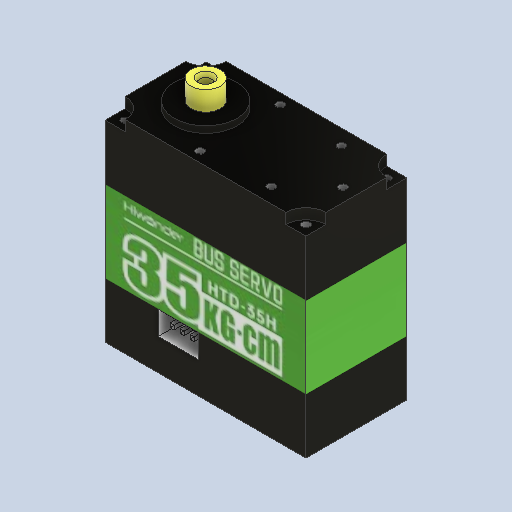
# Autodesk Inventor part: HTD-35H Servo
Saved by Autodesk Inventor 2023 (Build 270158000, 158)
## iProperties
Created: 2022-09-17
Part Number: HTD-35H Servo
Material: 일반
Document SubType Name: Modeling
Designer: 박동준
Density: 1 g/cm^3
Appearance: 기본값
Sheet Metal Rule: Default
품번: 6
Author: 박동준
Autodesk Inventor part; units mm, degrees
sketch "스케치1" plane through (0, 0, 0) normal (0, 0, 1) x (1, 0, 0)
  line L0 (-20.05, 20.25) -> (20.05, 20.25)
  line L1 (20.05, 20.25) -> (20.05, -20.25)
  line L2 (20.05, -20.25) -> (-20.05, -20.25)
  line L3 (-20.05, -20.25) -> (-20.05, 20.25)
  point P0 (0, 0)
  point P1 (0, 20.25)
  point P2 (-20.05, 0)
  dimension "d0" = 40.5
  dimension "d1" = 40.1
  constraints: 8 end point, 2 midpoint, 2 parallel, 1 horizontal, 1 horizontal alignment, 1 perpendicular, 1 vertical alignment
  measures "d0" distance of L2.end L0.start
  measures "d1" distance of L0.start L0.end
extrude "돌출1" add sketch "스케치1" along normal mid plane 20.14
sketch "스케치2" plane through (-20.05, 20.25, 10.07) normal (0, 1, 0) x (1, 0, 0)
  line L0 (16.9, 18.07) -> (16.9, 2.07) construction
  line L1 (0, 0) -> (40.1, 0) projected
  circle A0 centre (10, 10.07) radius 6.25
  line L2 (0, 20.14) -> (0, 0) projected
  point P0 (20.05, 10.07)
  point P1 (30.0912, 5.5667)
  point P2 (30.1, 12.7989)
  point P3 (37.0706, 12.5174)
  point P4 (16.9, 10.07)
  dimension "d4" = 16
  dimension "d6" = 13.2
  dimension "d7" = 12.5
  dimension "d8" = 6.9
  dimension "d9" = 10
  constraints: 2 end point, 2 horizontal alignment, 1 centre point, 1 midpoint, 1 perpendicular, 1 vertical alignment
  measures "d4" distance of L0.end L0.start
  measures "d6" horizontal distance of point (30.1, 12.799) L0.start
  measures "d7" diameter of A0
  measures "d8" horizontal distance of L0.start A0.centre
  measures "d9" distance from line of A0.centre L2
extrude "돌출2" add sketch "스케치2" along normal blind 1.3
sketch "스케치3" plane through (-20.05, -20.25, 10.07) normal (0, -1, 0) x (1, 0, 0)
  circle A0 centre (10, -10.07) radius 6.35
  line L0 (0, 0) -> (0, -20.14) projected
  point P0 (20.05, -10.07)
  dimension "d12" = 12.7
  dimension "d13" = 10
  constraints: 1 centre point, 1 horizontal alignment
  measures "d12" diameter of A0
  measures "d13" distance from line of A0.centre L0
extrude "돌출3" add sketch "스케치3" along normal blind 1.6
sketch "스케치4" plane through (-20.05, -20.25, 10.07) normal (0, -1, 0) x (1, 0, 0)
  circle A0 centre (10, -10.07) radius 6.35 construction
  line L0 (40.1, -20.14) -> (40.1, 0) construction
  line L1 (0, 0) -> (40.1, 0) construction
  line L2 (0, 0) -> (0, -20.14) construction
  line L3 (40.1, -20.14) -> (0, -20.14) construction
  line L4 (2.5, -2.545) -> (2.5, -17.595) construction
  line L5 (22.5, -2.545) -> (22.5, -17.595) construction
  line L6 (37.6, -2.545) -> (37.6, -17.595) construction
  point P0 (20.05, -10.07)
  point P1 (2.5, -10.07)
  point P2 (22.5, -10.07)
  point P3 (37.6, -10.07)
  dimension "d16" = 15.05
  dimension "d17" = 20
  dimension "d18" = 15.1
  dimension "d19" = 2.5
  constraints: 6 end point, 3 horizontal alignment, 3 midpoint, 2 vertical, 1 perpendicular
  measures "d16" distance of L4.end L4.start
  measures "d17" distance of L5.end L4.end
  measures "d18" distance of L6.end L5.end
  measures "d19" distance from line of L2 L4.end
hole "구멍1" at (-17.55, -20.25, 7.525) at (-17.55, -20.25, -7.525) at (2.45, -20.25, -7.525) at (2.45, -20.25, 7.525) at (17.55, -20.25, 7.525) at (17.55, -20.25, -7.525) direction (0, 1, 0) diameter 1.567 depth 10.6 thread size "M2x0.4" class "6H" standard "ISO Metric profile"
sketch "스케치5" plane through (0, 0, 10.07) normal (0, 0, 1) x (1, 0, 0)
  line L0 (-9.45, -9.25) -> (-1.45, -9.25)
  line L1 (-1.45, -9.25) -> (-1.45, -13.95)
  line L2 (-1.45, -13.95) -> (-9.45, -13.95)
  line L3 (-9.45, -13.95) -> (-9.45, -9.25)
  line L4 (-20.05, -20.25) -> (20.05, -20.25) projected
  line L5 (20.05, -20.25) -> (20.05, 20.25) projected
  point P0 (0, 0)
  dimension "d27" = 8
  dimension "d28" = 11
  dimension "d37" = 4.7
  dimension "d38" = 21.5
  constraints: 8 end point, 2 parallel, 1 horizontal, 1 perpendicular
  measures "d27" distance of L1.end L2.end
  measures "d28" distance between parallel lines of L0 L4
  measures "d37" distance of L0.end L1.end
  measures "d38" distance between parallel lines of L5 L1
extrude "돌출4" cut sketch "스케치5" against normal blind 5
sketch "스케치6" plane through (-10.05, -21.85, 0) normal (0, -1, 0) x (1, 0, 0)
  circle A0 centre (0, 0) radius 6.35 projected
  circle A1 centre (0, 0) radius 3
  point P0 (10.05, 0)
  dimension "d31" = 6
  constraints: 1 centre point, 1 coincident
  measures "d31" diameter of A1
extrude "돌출5" add sketch "스케치6" along normal blind 4.3 contours A1
sketch "스케치7" plane through (-10.05, -26.15, 0) normal (0, -1, 0) x (1, 0, 0)
  circle A0 centre (0, 0) radius 3 projected
  circle A1 centre (0, 0) radius 1.5
  point P0 (10.05, 0)
  dimension "d34" = 3
  constraints: 1 centre point, 1 coincident
  measures "d34" diameter of A1
extrude "돌출6" cut sketch "스케치7" against normal blind 8 contours A1
sketch "스케치8" plane through (-20.05, -20.25, 10.07) normal (-1, 0, 0) x (0, 0, 1)
  line L0 (0, 0) -> (-20.14, 0) construction
  line L1 (0, 40.5) -> (0, 0) construction
  line L2 (-20.14, 40.5) -> (0, 40.5) construction
  line L3 (-20.14, 0) -> (-20.14, 40.5) construction
  line L4 (-14.07, 11) -> (-6.07, 11)
  line L5 (-6.07, 11) -> (-6.07, 6.3)
  line L6 (-6.07, 6.3) -> (-14.07, 6.3)
  line L7 (-14.07, 6.3) -> (-14.07, 11)
  point P0 (-10.07, 20.25)
  point P1 (-10.07, 11)
  dimension "d39" = 8
  dimension "d40" = 4.7
  dimension "d41" = 11
  constraints: 8 end point, 2 parallel, 1 horizontal, 1 midpoint, 1 perpendicular, 1 vertical alignment
  measures "d39" distance of L5.end L6.end
  measures "d40" distance of L4.end L5.end
  measures "d41" distance between parallel lines of L0 L4
extrude "돌출7" cut sketch "스케치8" against normal blind 5
sketch "스케치9" plane through (0, 0, -10.07) normal (0, 0, -1) x (-1, 0, 0)
  line L0 (1.45, -9.25) -> (9.45, -9.25)
  line L1 (9.45, -9.25) -> (9.45, -13.95)
  line L2 (9.45, -13.95) -> (1.45, -13.95)
  line L3 (1.45, -13.95) -> (1.45, -9.25)
  line L4 (-20.05, -20.25) -> (20.05, -20.25) projected
  line L5 (-20.05, 20.25) -> (-20.05, -20.25) projected
  point P0 (0, 0)
  dimension "d44" = 8
  dimension "d45" = 4.7
  dimension "d46" = 11
  dimension "d47" = 21.5
  constraints: 8 end point, 2 parallel, 1 horizontal, 1 perpendicular
  measures "d44" distance of L1.end L2.end
  measures "d45" distance of L0.end L1.end
  measures "d46" distance between parallel lines of L4 L0
  measures "d47" distance between parallel lines of L5 L3
extrude "돌출8" cut sketch "스케치9" against normal blind 5
sketch "스케치10" plane through (-20.05, 20.25, 10.07) normal (0, 1, 0) x (1, 0, 0)
  circle A0 centre (10, 10.07) radius 6.25 projected
  line L0 (16.9, 18.07) -> (16.9, 2.07) construction
  line L1 (30.12, 17.07) -> (30.12, 3.07) construction
  point P0 (20.05, 10.07)
  point P1 (37.42, 10.07)
  point P2 (16.9, 10.07)
  point P3 (30.12, 10.07)
  dimension "d50" = 6.9
  dimension "d51" = 13.22
  dimension "d52" = 16
  dimension "d53" = 7.3
  dimension "d165" = 14
  constraints: 4 end point, 3 horizontal alignment, 2 midpoint, 2 vertical, 2 vertical alignment
  measures "d50" horizontal distance of L0.start A0.centre
  measures "d51" horizontal distance of L1.start L0.start
  measures "d52" distance of L0.end L0.start
  measures "d53" horizontal distance of L1.start point (37.42, 10.07)
  measures "d165" distance of L1.end L1.start
sketch "스케치11" plane through (0, 0, 0) normal (0, 0, 1) x (1, 0, 0)
  line L0 (-3.8, 21.55) -> (-16.3, 21.55) projected
  line L1 (-16.3, 20.25) -> (-3.8, 20.25) projected
  line L2 (-3.8, 21.55) -> (-16.3, 21.55) projected
  line L3 (-10.05, 21.55) -> (-10.05, 26.55)
  line L4 (-8.85, 24.65) -> (-8.425, 25.45)
  line L5 (-8.425, 25.45) -> (-7.125, 25.45)
  line L6 (-7.125, 25.45) -> (-7.125, 21.55)
  line L7 (-8.85, 24.65) -> (-8.85, 21.55)
  line L8 (-8.85, 21.55) -> (-7.125, 21.55)
  point P0 (0, 0)
  dimension "d54" = 5
  dimension "d55" = 5.85
  dimension "d56" = 2.4
  dimension "d57" = 1.3
  dimension "d58" = 0.8
  dimension "d59" = 3.9
  constraints: 12 end point, 2 perpendicular, 2 point on line, 1 collinear, 1 horizontal, 1 midpoint, 1 vertical
  measures "d54" distance of L3.start L3.end
  measures "d55" diameter of L6 L3
  measures "d56" diameter of L7 L3
  measures "d57" distance of L4.end L5.end
  measures "d58" distance from line of L4.start L5
  measures "d59" distance of L5.end L6.end
revolve "회전1" add sketch "스케치11" angle 360 about axis through (-10.05, 21.55, 0) along (0, 1, 0)
sketch "스케치12" plane through (0, 0, 5.07) normal (0, 0, 1) x (1, 0, 0)
  line L0 (-5.85, -11.2) -> (-5.05, -11.2)
  line L1 (-5.05, -11.2) -> (-5.05, -12)
  line L2 (-5.05, -12) -> (-5.85, -12)
  line L3 (-5.85, -12) -> (-5.85, -11.2)
  line L4 (-1.45, -13.95) -> (-9.45, -13.95) projected
  line L5 (-1.45, -9.25) -> (-1.45, -13.95) projected
  line L6 (-9.45, -9.25) -> (-1.45, -9.25) projected
  line L7 (-9.45, -13.95) -> (-9.45, -9.25) projected
  line L8 (-9.45, -13.95) -> (-9.45, -9.25) projected
  line L9 (-9.45, -9.25) -> (-1.45, -9.25) projected
  line L10 (-7.85, -11.2) -> (-7.05, -11.2)
  line L11 (-7.85, -12) -> (-7.85, -11.2)
  line L12 (-7.05, -12) -> (-7.85, -12)
  line L13 (-7.05, -11.2) -> (-7.05, -12)
  line L14 (-3.85, -11.2) -> (-3.05, -11.2)
  line L15 (-3.85, -12) -> (-3.85, -11.2)
  line L16 (-3.05, -12) -> (-3.85, -12)
  line L17 (-3.05, -11.2) -> (-3.05, -12)
  line L18 (-5.85, -11.2) -> (-5.05, -11.2)
  line L19 (-5.85, -12) -> (-5.85, -11.2)
  line L20 (-5.05, -12) -> (-5.85, -12)
  line L21 (-5.05, -11.2) -> (-5.05, -12)
  point P0 (0, 0)
  point P1 (-9.45, -11.6)
  point P2 (-5.85, -11.6)
  point P3 (-9.45, -11.6)
  point P4 (-5.45, -9.25)
  point P5 (-5.45, -11.2)
  point P6 (-7.45, -11.2)
  point P7 (-7.85, -11.6)
  point P8 (-3.45, -11.2)
  point P9 (-3.85, -11.6)
  point P10 (-5.45, -11.2)
  point P11 (-5.85, -11.6)
  dimension "d61" = 0.8
  dimension "d62" = 0.8
  dimension "d65" = 2
  dimension "d68" = 2
  constraints: 32 end point, 5 midpoint, 3 horizontal, 2 parallel, 1 horizontal alignment, 1 perpendicular, 1 vertical alignment, 30 other
  measures "d61" distance of L0.start L0.end
  measures "d62" distance of L0.end L1.end
  measures "d65" distance of L0.start L10.start
  measures "d68" distance of L0.start L14.start
extrude "돌출9" add sketch "스케치12" along normal blind 4.5 contours L0 L1 L2 L3 | L10 L13 L12 L11 | L14 L17 L16 L15
sketch "스케치13" plane through (-15.05, -20.25, 10.07) normal (-1, 0, 0) x (0, 0, 1)
  line L0 (-14.07, 11) -> (-6.07, 11) projected
  line L1 (-14.07, 6.3) -> (-14.07, 11) projected
  line L2 (-10.47, 9.05) -> (-9.67, 9.05)
  line L3 (-9.67, 9.05) -> (-9.67, 8.25)
  line L4 (-9.67, 8.25) -> (-10.47, 8.25)
  line L5 (-10.47, 8.25) -> (-10.47, 9.05)
  line L6 (-8.47, 9.05) -> (-7.67, 9.05)
  line L7 (-7.67, 9.05) -> (-7.67, 8.25)
  line L8 (-7.67, 8.25) -> (-8.47, 8.25)
  line L9 (-8.47, 8.25) -> (-8.47, 9.05)
  line L10 (-12.47, 9.05) -> (-11.67, 9.05)
  line L11 (-11.67, 9.05) -> (-11.67, 8.25)
  line L12 (-11.67, 8.25) -> (-12.47, 8.25)
  line L13 (-12.47, 8.25) -> (-12.47, 9.05)
  line L14 (-10.47, 9.05) -> (-9.67, 9.05)
  line L15 (-9.67, 9.05) -> (-9.67, 8.25)
  line L16 (-9.67, 8.25) -> (-10.47, 8.25)
  line L17 (-10.47, 8.25) -> (-10.47, 9.05)
  point P0 (-10.07, 20.25)
  point P1 (-10.07, 11)
  point P2 (-10.07, 9.05)
  point P3 (-14.07, 8.65)
  point P4 (-10.47, 8.65)
  point P5 (-8.07, 9.05)
  point P6 (-8.47, 8.65)
  point P7 (-12.07, 9.05)
  point P8 (-12.47, 8.65)
  point P9 (-10.07, 9.05)
  point P10 (-10.47, 8.65)
  dimension "d76" = 0.8
  dimension "d77" = 0.8
  dimension "d80" = 2
  dimension "d83" = 2
  constraints: 32 end point, 4 midpoint, 3 horizontal, 2 parallel, 1 horizontal alignment, 1 perpendicular, 1 vertical alignment, 30 other
  measures "d76" distance of L3.end L4.end
  measures "d77" distance of L2.end L3.end
  measures "d80" distance of L2.start L6.start
  measures "d83" distance of L2.start L10.start
extrude "돌출10" add sketch "스케치13" along normal blind 4.5
sketch "스케치14" plane through (0, 0, -5.07) normal (0, 0, -1) x (-1, 0, 0)
  line L0 (9.45, -13.95) -> (1.45, -13.95) projected
  line L1 (9.45, -9.25) -> (9.45, -13.95) projected
  line L2 (1.45, -9.25) -> (9.45, -9.25) projected
  line L3 (1.45, -13.95) -> (1.45, -9.25) projected
  line L4 (5.05, -11.2) -> (5.85, -11.2)
  line L5 (5.85, -11.2) -> (5.85, -12)
  line L6 (5.85, -12) -> (5.05, -12)
  line L7 (5.05, -12) -> (5.05, -11.2)
  line L8 (1.45, -9.25) -> (9.45, -9.25) projected
  line L9 (1.45, -13.95) -> (1.45, -9.25) projected
  line L10 (7.05, -11.2) -> (7.85, -11.2)
  line L11 (7.85, -11.2) -> (7.85, -12)
  line L12 (7.85, -12) -> (7.05, -12)
  line L13 (7.05, -12) -> (7.05, -11.2)
  line L14 (3.05, -11.2) -> (3.85, -11.2)
  line L15 (3.85, -11.2) -> (3.85, -12)
  line L16 (3.85, -12) -> (3.05, -12)
  line L17 (3.05, -12) -> (3.05, -11.2)
  line L18 (5.05, -11.2) -> (5.85, -11.2)
  line L19 (5.85, -11.2) -> (5.85, -12)
  line L20 (5.85, -12) -> (5.05, -12)
  line L21 (5.05, -12) -> (5.05, -11.2)
  point P0 (0, 0)
  point P1 (5.45, -9.25)
  point P2 (5.45, -11.2)
  point P3 (1.45, -11.6)
  point P4 (5.05, -11.6)
  point P5 (7.45, -11.2)
  point P6 (7.05, -11.6)
  point P7 (3.45, -11.2)
  point P8 (3.05, -11.6)
  point P9 (5.45, -11.2)
  point P10 (5.05, -11.6)
  dimension "d88" = 0.8
  dimension "d89" = 0.8
  dimension "d92" = 2
  dimension "d95" = 2
  constraints: 32 end point, 4 midpoint, 3 horizontal, 2 parallel, 1 horizontal alignment, 1 perpendicular, 1 vertical alignment, 30 other
  measures "d88" distance of L5.end L6.end
  measures "d89" distance of L4.end L5.end
  measures "d92" distance of L4.start L10.start
  measures "d95" distance of L4.start L14.start
extrude "돌출11" add sketch "스케치14" along normal blind 4.5 contours L4 L5 L6 L7 | L10 L11 L12 L13 | L14 L15 L16 L17
chamfer "모따기2" distance 0.25 angle 45 36 edges at (-3.85, -11.6, -9.57) (-3.45, -12, -9.57) (-3.05, -11.6, -9.57) (-3.45, -11.2, -9.57) (-5.05, -11.6, -9.57) (-5.45, -12, -9.57) (-5.85, -11.6, -9.57) (-5.45, -11.2, -9.57) (-7.45, -12, -9.57) (-7.85, -11.6, -9.57) (-7.45, -11.2, -9.57) (-7.05, -11.6, -9.57) (-19.55, -11.2, -2) (-19.55, -11.6, -2.4) (-19.55, -12, -2) (-19.55, -11.6, -1.6) (-19.55, -11.6, -0.4) (-19.55, -12, 0) (-19.55, -11.6, 0.4) (-19.55, -11.2, 0) (-19.55, -11.6, 1.6) (-19.55, -12, 2) (-19.55, -11.6, 2.4) (-19.55, -11.2, 2) (-7.45, -12, 9.57) (-7.05, -11.6, 9.57) (-7.45, -11.2, 9.57) (-7.85, -11.6, 9.57) (-5.45, -12, 9.57) (-5.05, -11.6, 9.57) (-5.45, -11.2, 9.57) (-5.85, -11.6, 9.57) (-3.85, -11.6, 9.57) (-3.45, -12, 9.57) (-3.05, -11.6, 9.57) (-3.45, -11.2, 9.57)
sketch "스케치15" plane through (-20.05, 20.25, 10.07) normal (0, 1, 0) x (1, 0, 0)
  line L0 (40.1, 20.14) -> (40.1, 0) construction
  line L1 (40.1, 20.14) -> (0, 20.14) construction
  arc A0 (36.1, 20.14) -> (40.1, 16.14) centre (40.1, 20.14) ccw
  line L2 (20.05, 25.8299) -> (20.05, -7.9566) construction
  line L3 (-11.132, 10.07) -> (46.3256, 10.07) construction
  line L4 (36.1, 20.14) -> (40.1, 20.14)
  line L5 (40.1, 20.14) -> (40.1, 16.14)
  arc A1 (0, 16.14) -> (4, 20.14) centre (0, 20.14) ccw
  arc A2 (40.1, 4) -> (36.1, 0) centre (40.1, 0) ccw
  arc A3 (4, 0) -> (0, 4) centre (0, 0) ccw
  line L6 (0, 0) -> (0, 20.14) projected
  line L7 (0, 16.14) -> (0, 20.14)
  line L8 (0, 20.14) -> (4, 20.14)
  line L9 (0, 0) -> (40.1, 0) projected
  line L10 (0, 0) -> (0, 4)
  line L11 (0, 0) -> (4, 0)
  line L12 (40.1, 0) -> (36.1, 0)
  line L13 (40.1, 0) -> (40.1, 4)
  point P0 (20.05, 10.07)
  dimension "d103" = 4
  constraints: 20 end point, 8 point on circle, 7 symmetric about line, 4 centre point, 4 collinear, 3 perpendicular, 2 vertical, 1 horizontal, 1 point on line, 3 other
  measures "d103" radius of A0
extrude "돌출12" cut sketch "스케치15" against normal blind 2.1
sketch "스케치16" plane through (-20.05, 18.15, 10.07) normal (0, 1, 0) x (1, 0, 0)
  line L0 (0, 20.14) -> (4, 20.14) projected
  line L1 (36.1, 20.14) -> (40.1, 20.14) projected
  line L2 (40.1, 0) -> (36.1, 0) projected
  line L3 (4, 0) -> (0, 0) projected
  line L4 (0, 16.14) -> (0, 20.14) projected
  line L5 (0, 0) -> (0, 4) projected
  line L6 (40.1, 4) -> (40.1, 0) projected
  line L7 (40.1, 20.14) -> (40.1, 16.14) projected
  point P0 (20.05, 10.07)
  point P1 (38.1, 18.14)
  point P2 (38.1, 2)
  point P3 (2, 2)
  point P4 (2, 18.14)
  point P5 (2, 20.14)
  point P6 (38.1, 20.14)
  point P7 (38.1, 0)
  point P8 (2, 0)
  point P9 (0, 18.14)
  point P10 (0, 2)
  point P11 (40.1, 2)
  point P12 (40.1, 18.14)
  constraints: 8 midpoint, 4 horizontal alignment, 4 vertical alignment
hole "구멍2" at (18.05, 18.15, 8.07) at (18.05, 18.15, -8.07) at (-18.05, 18.15, -8.07) at (-18.05, 18.15, 8.07) direction (0, -1, 0) diameter 1.567 depth 10.6 thread size "M2x0.4" class "6H" standard "ISO Metric profile"
sketch "스케치17" plane through (0, 0, 10.07) normal (0, 0, 1) x (1, 0, 0)
  line L0 (-19.75, 6.866) -> (19.75, 6.866) construction
  line L1 (19.75, 6.866) -> (19.75, -9.25) construction
  line L2 (19.75, -9.25) -> (-19.75, -9.25) construction
  line L3 (-19.75, -9.25) -> (-19.75, 6.866) construction
  line L4 (-20.05, 18.15) -> (-20.05, -20.25) construction
  line L5 (-9.45, -9.25) -> (-1.45, -9.25) projected
  line L6 (-20.05, -20.25) -> (20.05, -20.25) construction
  point P0 (0, 0)
  point P1 (0, -9.25)
  point P2 (0, -20.25)
  dimension "d122" = 0
  dimension "d124" = 16.116
  constraints: 2 midpoint, 1 vertical, 1 vertical alignment, 2 other
  measures "d122" distance between parallel lines of L5 L2
  measures "d124" distance of L0.end L1.end
ref_plane "작업 평면1" through (0, 0, 40) normal (0, 0, 1) x (1, 0, 0)
sketch "스케치19" plane through (0, 0, 40) normal (0, 0, 1) x (1, 0, 0)
  line L0 (-20.05, 7.1108) -> (20.05, 7.1108) construction
  line L1 (20.05, 7.1108) -> (20.05, -9.25) construction
  line L2 (20.05, -9.25) -> (-20.05, -9.25) construction
  line L3 (-20.05, -9.25) -> (-20.05, 7.1108) construction
  line L4 (20.05, -20.25) -> (20.05, 18.15) projected
  line L5 (-9.45, -9.25) -> (-1.45, -9.25) projected
  point P0 (0, 0)
  point P1 (20.05, -1.0696)
  point P2 (20.05, -1.05)
  dimension "d145" = 40.1
  dimension "d152" = 0
  constraints: 2 midpoint, 1 vertical alignment, 2 other
  measures "d145" distance of L1.end L2.end
  measures "d152" distance between parallel lines of L5 L2
decal "전사1"
ref_plane "작업 평면2" through (0, 0, -70.57) normal (0, 0, -1) x (-1, 0, 0)
sketch "스케치20" plane through (0, 0, -70.57) normal (0, 0, -1) x (-1, 0, 0)
  line L0 (-20.05, 7.1108) -> (20.05, 7.1108) construction
  line L1 (20.05, 7.1108) -> (20.05, -9.25) construction
  line L2 (20.05, -9.25) -> (-20.05, -9.25) construction
  line L3 (-20.05, -9.25) -> (-20.05, 7.1108) construction
  line L4 (20.05, -20.25) -> (20.05, 18.15) projected
  line L5 (1.45, -9.25) -> (9.45, -9.25) projected
  point P0 (0, 0)
  point P1 (20.05, -1.0696)
  point P2 (20.05, -1.05)
  dimension "d157" = 40.1
  dimension "d162" = 0
  constraints: 2 midpoint, 1 vertical alignment, 2 other
  measures "d157" distance of L1.end L2.end
  measures "d162" distance between parallel lines of L5 L2
decal "전사2"
hole "구멍3" at (-3.15, 20.25, 8) at (-3.15, 20.25, -8) at (10.07, 20.25, -7) at (10.07, 20.25, 7) at (17.37, 20.25, 0) direction (0, -1, 0) diameter 1.567 depth 10.6 thread size "M2x0.4" class "6H" standard "ISO Metric profile"
ref_plane "작업 평면3" through (56.3, -20.25, 10.07) normal (1, 0, 0) x (0, 0, -1)
sketch "스케치21" plane through (56.3, -20.25, 10.07) normal (1, 0, 0) x (0, 0, -1)
  line L0 (-0.1058, 27.2499) -> (20.14, 27.2499) construction
  line L1 (20.14, 27.2499) -> (20.14, 11) construction
  line L2 (20.14, 11) -> (-0.1058, 11) construction
  line L3 (-0.1058, 11) -> (-0.1058, 27.2499) construction
  line L4 (20.14, 38.4) -> (20.14, 0) projected
  line L5 (20.14, 0) -> (0, 0) projected
  point P0 (10.07, 20.25)
  point P1 (20.14, 19.125)
  point P2 (20.14, 19.2)
  dimension "d184" = 11
  constraints: 2 midpoint, 1 vertical alignment, 2 other
  measures "d184" distance between parallel lines of L5 L2
decal "전사3"
ref_plane "작업 평면4" through (-52.55, -20.25, -10.07) normal (-1, 0, 0) x (0, 0, 1)
sketch "스케치22" plane through (-52.55, -20.25, -10.07) normal (-1, 0, 0) x (0, 0, 1)
  line L0 (0.0342, 27.1376) -> (20.14, 27.1376) construction
  line L1 (20.14, 27.1376) -> (20.14, 11) construction
  line L2 (20.14, 11) -> (0.0342, 11) construction
  line L3 (0.0342, 11) -> (0.0342, 27.1376) construction
  line L4 (20.14, 38.4) -> (20.14, 0) projected
  line L5 (6.07, 11) -> (14.07, 11) projected
  point P0 (10.07, 20.25)
  dimension "d187" = 20.1058
  dimension "d188" = 0
  dimension "d190" = 0
  constraints: 2 other
  measures "d187" distance of L1.end L2.end
  measures "d188" distance between parallel lines of L4 L1
  measures "d190" distance between parallel lines of L5 L2
decal "전사4"
equation "\"TransitionRadius\" = BendRadius"
equation "\"BendRadius\" = 3.048"
